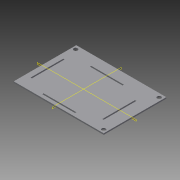
# Autodesk Inventor part: mount_plate
Saved by Autodesk Inventor 2015 SP1 (Build 190203100, 203)
## iProperties
Created: 2016-08-02
Part Number: mount_plate
Material: Generic
Document SubType Name: Modeling
Designer: polidorop
Density: 1 g/cm^3
Appearance: Default
Author: polidorop
Autodesk Inventor part; units mm, degrees
ref_plane "YZ Plane" through (0, 0, 0) normal (1, 0, 0) x (0, 1, 0)
ref_plane "XZ Plane" through (0, 0, 0) normal (0, 1, 0) x (-1, 0, 0)
ref_plane "XY Plane" through (0, 0, 0) normal (0, 0, 1) x (1, 0, 0)
sketch "Sketch2" plane through (0, 0, 0) normal (0, 0, 1) x (1, 0, 0)
  circle A0 centre (5, 90) radius 3
  circle A1 centre (133, 5) radius 3
  circle A2 centre (133, 90) radius 3
  line L0 (0, 0) -> (138, 0)
  line L1 (138, 0) -> (138, 96)
  line L2 (138, 96) -> (0, 96)
  line L3 (0, 96) -> (0, 0)
  circle A3 centre (6, 20) radius 2
  circle A4 centre (6, 66) radius 2
  circle A5 centre (122, 40) radius 2
  constraints: 8 end point, 6 centre point, 4 equal radius, 2 perpendicular, 1 parallel
extrude "Extrusion2" add sketch "Sketch2" along normal mid plane 2 contours L3 L2 L1 L0 | A3 | A4 | A5
sketch "Sketch3" plane through (0, 0, 1) normal (0, 0, 1) x (1, 0, 0)
  circle A0 centre (6, 20) radius 2 construction
  circle A1 centre (6, 20) radius 0.5
  point P0 (0, 0)
  dimension "d4" = 1
  constraints: 1 centre point, 1 coincident
  measures "d4" diameter of A1
extrude "Extrusion3" [suppressed]
sketch "Sketch4" plane through (0, 0, 1) normal (0, 0, 1) x (1, 0, 0)
  circle A0 centre (6, 66) radius 2 projected
  circle A1 centre (6, 66) radius 0.5
  point P0 (0, 0)
  dimension "d7" = 1
  constraints: 1 centre point, 1 coincident
  measures "d7" diameter of A1
extrude "Extrusion4" [suppressed]
sketch "Sketch5" plane through (0, 0, 1) normal (0, 0, 1) x (1, 0, 0)
  circle A0 centre (122, 40) radius 2 projected
  circle A1 centre (122, 40) radius 0.5
  point P0 (0, 0)
  dimension "d10" = 1
  constraints: 1 centre point, 1 coincident
  measures "d10" diameter of A1
extrude "Extrusion5" [suppressed]
ref_plane "Work Plane1" through (64, 0, 1) normal (-1, 0, 0) x (0, 0, 1)
ref_plane "Work Plane2" through (0, 43, 1) normal (0, -1, 0) x (1, 0, 0)
sketch "Sketch7" plane through (0, 0, 1) normal (0, 0, 1) x (1, 0, 0)
  line L0 (39, 7) -> (89, 7)
  line L1 (89, 7) -> (89, 5)
  line L2 (89, 5) -> (39, 5)
  line L3 (39, 5) -> (39, 7)
  line L4 (64, -19.2) -> (64, 115.2) construction
  line L5 (165.6, 43) -> (-27.6, 43) construction
  line L6 (0, 0) -> (138, 0) projected
  line L7 (8, 68) -> (10, 68)
  line L8 (10, 68) -> (10, 18)
  line L9 (10, 18) -> (8, 18)
  line L10 (8, 18) -> (8, 68)
  line L11 (0, 96) -> (0, 0) projected
  line L12 (118, 68) -> (120, 68)
  line L13 (120, 68) -> (120, 18)
  line L14 (120, 18) -> (118, 18)
  line L15 (118, 18) -> (118, 68)
  line L16 (39, 80) -> (89, 80)
  line L17 (89, 80) -> (89, 78)
  line L18 (89, 78) -> (39, 78)
  line L19 (39, 78) -> (39, 80)
  point P0 (64, 7)
  point P1 (10, 43)
  point P2 (118, 43)
  point P3 (64, 78)
  dimension "d15" = 2
  dimension "d16" = 5
  dimension "d17" = 50
  dimension "d18" = 2
  dimension "d19" = 50
  dimension "d20" = 8
  dimension "d23" = 50
  dimension "d24" = 2
  dimension "d25" = 118
  dimension "d26" = 2
  dimension "d27" = 50
  dimension "d28" = 78
  constraints: 32 end point, 8 parallel, 4 horizontal, 4 midpoint, 4 perpendicular, 4 point on line
  measures "d15" distance of L2.end L0.start
  measures "d16" distance between parallel lines of L6 L2
  measures "d17" distance of L0.start L0.end
  measures "d18" distance of L8.end L9.end
  measures "d19" distance of L7.end L8.end
  measures "d20" distance between parallel lines of L11 L10
  measures "d23" distance of L12.end L13.end
  measures "d24" distance of L13.end L14.end
  measures "d25" distance from line of L15 L6.start
  measures "d26" distance of L16.end L17.end
  measures "d27" distance of L16.start L16.end
  measures "d28" distance from line of L6.start L18
extrude "Extrusion6" cut sketch "Sketch7" against normal through all
body "Solid2"
